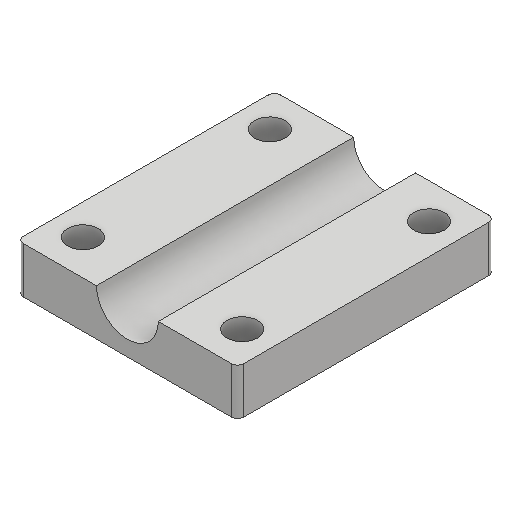
# Autodesk Inventor part: 3DP_ABS_X_Axis_Linear_Shaft_Clamp_Base
Saved by Autodesk Inventor 2026.1 (Build 301233000, 233)
## iProperties
Created: 2017-05-25
Part Number: 3DP_ABS_X_Axis_Linear_Shaft_Clamp_Base
Material: Ogólny
Document SubType Name: Modeling
Designer: Andrzej
Density: 1 g/cm^3
Appearance: Domyślna
Mass: 9.34713 g
Surface Area: 46.2811 cm^2
Volume: 9.34713 cm^3
Author: Andrzej
Autodesk Inventor part; units mm, degrees
ref_plane "YZ Plane" through (0, 0, 0) normal (1, 0, 0) x (0, 1, 0)
ref_plane "XZ Plane" through (0, 0, 0) normal (0, 1, 0) x (-1, 0, 0)
ref_plane "XY Plane" through (0, 0, 0) normal (0, 0, 1) x (1, 0, 0)
sketch "Szkic1" plane through (0, 0, 0) normal (0, 0, 1) x (1, 0, 0)
  line L0 (-10.3866, 5.557) -> (25.6134, 5.557)
  line L1 (25.6134, 5.557) -> (25.6134, -36.443)
  line L2 (25.6134, -36.443) -> (-10.3866, -36.443)
  line L3 (-10.3866, -36.443) -> (-10.3866, 5.557)
  point P0 (0, 0)
  point P1 (20.6134, -0.193)
  point P2 (20.6134, -30.693)
  point P3 (-5.3866, -0.193)
  point P4 (-5.3866, -30.693)
  dimension "d0" = 36
  dimension "d1" = 42
  dimension "d2" = 5
  dimension "d3" = 5
  dimension "d4" = 5
  dimension "d5" = 5
  dimension "d6" = 5.75
  dimension "d7" = 5.75
  dimension "d8" = 5.75
  dimension "d9" = 5.75
  constraints: 8 end point, 2 parallel, 1 horizontal, 1 perpendicular
  measures "d0" distance of L1.end L2.end
  measures "d1" distance of L0.end L1.end
  measures "d2" distance from line of L1 point (20.613, -0.193)
  measures "d3" distance from line of L1 point (20.613, -30.693)
  measures "d4" distance from line of L3 point (-5.387, -0.193)
  measures "d5" distance from line of L3 point (-5.387, -30.693)
  measures "d6" distance from line of L0 point (-5.387, -0.193)
  measures "d7" distance from line of L0 point (20.613, -0.193)
  measures "d8" distance from line of L2 point (20.613, -30.693)
  measures "d9" distance from line of L2 point (-5.387, -30.693)
extrude "Wyciągnięcie proste1" add sketch "Szkic1" along normal blind 7.55
hole "Otwór1" at (20.6134, -0.193, 0) at (20.6134, -30.693, 0) at (-5.3866, -0.193, 0) at (-5.3866, -30.693, 0) direction (0, 0, 1) diameter 5 end through all
sketch "Szkic2" plane through (-10.3866, -36.443, 0) normal (0, -1, 0) x (1, 0, 0)
  line L0 (36, 0) -> (0, 0) projected
  line L1 (36, 0) -> (36, 7.55) projected
  line L2 (0, 7.55) -> (36, 7.55) projected
  line L3 (0, 0) -> (0, 7.55) projected
  line L4 (36, 7.55) -> (0, 7.55) projected
  circle A0 centre (18, 7.55) radius 5.05
  point P0 (10.3866, 0)
  dimension "d19" = 36
  dimension "d20" = 18
  dimension "d21" = 10.1
  constraints: 1 centre point, 1 coincident, 1 midpoint
  measures "d19" distance between parallel lines of L1 L3
  measures "d20" distance from line of L3 point (18, 7.55)
  measures "d21" diameter of A0
extrude "Wyciągnięcie proste2" cut sketch "Szkic2" against normal through all contours A0 L2 | L2 A0
fillet "Zaokrąglenie1" radius 1 4 edges at (-10.3866, -36.443, 3.775) (-10.3866, 5.557, 3.775) (25.6134, -36.443, 3.775) (25.6134, 5.557, 3.775)
equation "\"d7\" = d6"
equation "\"d8\" = d7"
equation "\"d9\" = d6"
equation "\"d20\" = 0.5 * d19"
